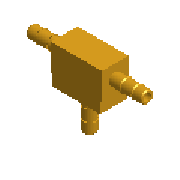
# Autodesk Inventor part: Tubo en T de unión 224 de Parker 224-6
Saved by Autodesk Inventor 2021 (Build 250183000, 183)
## iProperties
NAME: PIPING: Parker Union Tee 224
DATA: <meta><inlinegroups number="1" deflen="2.54"></inlinegroups><connections number="3"></connections><angles><a>3.14159265358979</a><a>1.57079632679489</a></angles></meta>
IsCustomPart: 0
Created: 2020-01-21
Part Number: Tubo en T de unión 224 de Parker 224-6
Material: Latón, amarillo claro
Description: Tubo en T de unión
Document SubType Name: Modeling
Standard: Parker
Designer: Admin
Manufacturer: Parker
Language: es-ES
Size Designation: 224-6
Categories: <MemberInstance><Categories><Category DisplayName="Tubo y tubería" InternalName="4347fa0f-2144-441d-94cd-e3e15c92b736" Mnemonic="TUBEANDPIPE"><CategoryParameter DisplayName="Número de conexiones" InternalName="04e9c83a-9e20-4a98-a7e1-e8abe87a2846" Mnemonic="NUM_CONNECTIONS"/><CategoryParameter DisplayName="Angles" InternalName="0e0e4fa4-3bd3-4656-a22e-4e07c8c476f8" Mnemonic="ANGLES"><CategoryParameter DisplayName="Angle" InternalName="9188ad83-1b16-48b4-8b0a-76ce729dafa7" Mnemonic="ANGLE"/></CategoryParameter><CategoryParameter DisplayName="Angles" InternalName="0e0e4fa4-3bd3-4656-a22e-4e07c8c476f8" Mnemonic="ANGLES"><CategoryParameter DisplayName="Angle" InternalName="9188ad83-1b16-48b4-8b0a-76ce729dafa7" Mnemonic="ANGLE"/></CategoryParameter><CategoryParameter DisplayName="Clave" InternalName="3da84699-049a-4bc2-a65a-6696b77c242f" Mnemonic="SKEY"/><CategoryParameter DisplayName="Descripción ISOGEN" InternalName="7aa3ba45-b821-4467-8584-f9e6f15f2a7d" Mnemonic="ISOGENDESC"/><CategoryParameter DisplayName="CÓDIGO-ARTÍCULO" InternalName="99cc3b15-24d9-4d38-aac7-792cfbc57acf" Mnemonic="ITEMCODE"/><CategoryParameter DisplayName="NombreDeComponente" InternalName="9c74ad13-48a1-45fe-b0f7-5447561f444a" Mnemonic="NAMEOFCOMPONENT"/><CategoryParameter DisplayName="GruposEnLínea" InternalName="d60be647-bc43-4c18-a13f-9fe4115f8e64" Mnemonic="INLINEGROUPS"/><Category DisplayName="Accesorios" InternalName="ed6b26c4-72b8-4f31-9b63-f85ae8f932e4" Mnemonic="FITTINGS"><CategoryParameter DisplayName="Connections" InternalName="dbd721e8-e885-4eea-9011-b5acfd9f61de" Mnemonic="FIT_CONNECTIONS"><CategoryParameter DisplayName="Tamaño de tubería de conicidencia mín." InternalName="11f51b32-3e37-4310-abf7-f1318a1fd129" Mnemonic="MNMPS"/><CategoryParameter DisplayName="EngraneMáx" InternalName="34fdf028-8797-436e-ba07-ca3dee15bd9b" Mnemonic="MAXENGAGEMENT"/><CategoryParameter DisplayName="TamañoNominal" InternalName="3f94edc7-e459-48db-8f02-8eebf8cffccd" Mnemonic="NS"/><CategoryParameter DisplayName="NombreVisualización" InternalName="50f521dd-e050-43f7-9895-6b30ea7ed42e" Mnemonic="DISPLAYNAME"/><CategoryParameter DisplayName="Cortar tubería de coincidencia" InternalName="53a63a6e-53d8-4ca9-8880-037731d1cceb" Mnemonic="CMP"/><CategoryParameter DisplayName="Género neutro" InternalName="628bd5f1-acad-44e2-9d91-af996ab74fc2" Mnemonic="NEUTRAL"/><CategoryParameter DisplayName="EngraneMín [% de EngraneMáx]" InternalName="7ec1bde5-73f0-45b1-98d8-365a6c67f8ad" Mnemonic="MINENGAGEMENT"/><CategoryParameter DisplayName="Fijo" InternalName="9142902a-6a8a-446d-9eb8-4b7ce7d245ef" Mnemonic="FIXED"/><CategoryParameter DisplayName="Hembra" InternalName="b366bcb5-a500-4bad-84bb-22f956216d69" Mnemonic="FEMALE"/><CategoryParameter DisplayName="DirecciónGiro" InternalName="d55dedc0-f14a-4283-86b4-a4eeb253c8aa" Mnemonic="FLIPDIRECTION"/><CategoryParameter DisplayName="NúmeroPlanificación" InternalName="d6161c62-eb59-4495-a086-874847c10866" Mnemonic="SN"/><CategoryParameter DisplayName="TratamientoFinal" InternalName="d7f11516-3374-45ca-b1c7-4b2d63244ae2" Mnemonic="ENDTREATMENT"/><CategoryParameter DisplayName="Tamaño de tubería de conicidencia máx." InternalName="e73ef66b-c04b-45ac-9b32-f712653e25ee" Mnemonic="MXMPS"/></CategoryParameter><CategoryParameter DisplayName="Connections" InternalName="dbd721e8-e885-4eea-9011-b5acfd9f61de" Mnemonic="FIT_CONNECTIONS"><CategoryParameter DisplayName="Tamaño de tubería de conicidencia mín." InternalName="11f51b32-3e37-4310-abf7-f1318a1fd129" Mnemonic="MNMPS"/><CategoryParameter DisplayName="EngraneMáx" InternalName="34fdf028-8797-436e-ba07-ca3dee15bd9b" Mnemonic="MAXENGAGEMENT"/><CategoryParameter DisplayName="TamañoNominal" InternalName="3f94edc7-e459-48db-8f02-8eebf8cffccd" Mnemonic="NS"/><CategoryParameter DisplayName="NombreVisualización" InternalName="50f521dd-e050-43f7-9895-6b30ea7ed42e" Mnemonic="DISPLAYNAME"/><CategoryParameter DisplayName="Cortar tubería de coincidencia" InternalName="53a63a6e-53d8-4ca9-8880-037731d1cceb" Mnemonic="CMP"/><CategoryParameter DisplayName="Género neutro" InternalName="628bd5f1-acad-44e2-9d91-af996ab74fc2" Mnemonic="NEUTRAL"/><CategoryParameter DisplayName="EngraneMín [% de EngraneMáx]" InternalName="7ec1bde5-73f0-45b1-98d8-365a6c67f8ad" Mnemonic="MINENGAGEMENT"/><CategoryParameter DisplayName="Fijo" InternalName="9142902a-6a8a-446d-9eb8-4b7ce7d245ef" Mnemonic="FIXED"/><CategoryParameter DisplayName="Hembra" InternalName="b366bcb5-a500-4bad-84bb-22f956216d69" Mnemonic="FEMALE"/><CategoryParameter DisplayName="DirecciónGiro" InternalName="d55dedc0-f14a-4283-86b4-a4eeb253c8aa" Mnemonic="FLIPDIRECTION"/><CategoryParameter DisplayName="NúmeroPlanificación" InternalName="d6161c62-eb59-4495-a086-874847c10866" Mnemonic="SN"/><CategoryParameter DisplayName="TratamientoFinal" InternalName="d7f11516-3374-45ca-b1c7-4b2d63244ae2" Mnemonic="ENDTREATMENT"/><CategoryParameter DisplayName="Tamaño de tubería de conicidencia máx." InternalName="e73ef66b-c04b-45ac-9b32-f712653e25ee" Mnemonic="MXMPS"/></CategoryParameter><CategoryParameter DisplayName="Connections" InternalName="dbd721e8-e885-4eea-9011-b5acfd9f61de" Mnemonic="FIT_CONNECTIONS"><CategoryParameter DisplayName="Tamaño de tubería de conicidencia mín." InternalName="11f51b32-3e37-4310-abf7-f1318a1fd129" Mnemonic="MNMPS"/><CategoryParameter DisplayName="EngraneMáx" InternalName="34fdf028-8797-436e-ba07-ca3dee15bd9b" Mnemonic="MAXENGAGEMENT"/><CategoryParameter DisplayName="TamañoNominal" InternalName="3f94edc7-e459-48db-8f02-8eebf8cffccd" Mnemonic="NS"/><CategoryParameter DisplayName="NombreVisualización" InternalName="50f521dd-e050-43f7-9895-6b30ea7ed42e" Mnemonic="DISPLAYNAME"/><CategoryParameter DisplayName="Cortar tubería de coincidencia" InternalName="53a63a6e-53d8-4ca9-8880-037731d1cceb" Mnemonic="CMP"/><CategoryParameter DisplayName="Género neutro" InternalName="628bd5f1-acad-44e2-9d91-af996ab74fc2" Mnemonic="NEUTRAL"/><CategoryParameter DisplayName="EngraneMín [% de EngraneMáx]" InternalName="7ec1bde5-73f0-45b1-98d8-365a6c67f8ad" Mnemonic="MINENGAGEMENT"/><CategoryParameter DisplayName="Fijo" InternalName="9142902a-6a8a-446d-9eb8-4b7ce7d245ef" Mnemonic="FIXED"/><CategoryParameter DisplayName="Hembra" InternalName="b366bcb5-a500-4bad-84bb-22f956216d69" Mnemonic="FEMALE"/><CategoryParameter DisplayName="DirecciónGiro" InternalName="d55dedc0-f14a-4283-86b4-a4eeb253c8aa" Mnemonic="FLIPDIRECTION"/><CategoryParameter DisplayName="NúmeroPlanificación" InternalName="d6161c62-eb59-4495-a086-874847c10866" Mnemonic="SN"/><CategoryParameter DisplayName="TratamientoFinal" InternalName="d7f11516-3374-45ca-b1c7-4b2d63244ae2" Mnemonic="ENDTREATMENT"/><CategoryParameter DisplayName="Tamaño de tubería de conicidencia máx." InternalName="e73ef66b-c04b-45ac-9b32-f712653e25ee" Mnemonic="MXMPS"/></CategoryParameter><Category DisplayName="Tubos en T" InternalName="63457372-9f68-4568-9fa2-68fa0de1b1dd" Mnemonic="Tee"/></Category></Category><Category DisplayName="TipoDatos" InternalName="23b78d0f-2648-40c6-8793-ca6db495c9e8" Mnemonic="DATATYPE"><CategoryParameter DisplayName="NombreVisualización" InternalName="05415f3d-3907-474b-a020-eb9d644f4cf3" Mnemonic="DISPLAYNAME"/><CategoryParameter DisplayName="Estándar" InternalName="0c0a119c-1e12-4c84-803f-101930972f5e" Mnemonic="STANDARD"/><CategoryParameter DisplayName="Descripción" InternalName="13903e3d-64b1-4950-80da-f627842ea37f" Mnemonic="DESCRIPTION"/><CategoryParameter DisplayName="Designación" InternalName="2675968c-4ce5-49e0-a4f5-552d29089031" Mnemonic="DESIGNATION"/><CategoryParameter DisplayName="Fila por defecto" InternalName="2af9ec52-faaa-4026-b378-f9fa4afca842" Mnemonic="DEFAULTROW"/><CategoryParameter DisplayName="Nombre de carpeta" InternalName="3f06958e-8713-4116-9be7-ed6184ecc97b" Mnemonic="FOLDERNAME"/><CategoryParameter DisplayName="Guid de revisión" InternalName="45a75005-10b1-4dfc-8d6d-dfe629f0b93c" Mnemonic="REVISIONGUID"/><CategoryParameter DisplayName="NombreArchivo" InternalName="8b46a4cc-9585-4fed-90c3-899f57e09a73" Mnemonic="FILENAME"/><CategoryParameter DisplayName="OrgEstand" InternalName="8f5914e1-4693-403f-8ab5-d37768198c9d" Mnemonic="STDSORG"/><CategoryParameter DisplayName="Versión de familia" InternalName="914462f6-6e19-4b14-ba84-155b9680b1d0" Mnemonic="FAMILYREVISION"/><CategoryParameter DisplayName="Revisión de Norma" InternalName="91d5a463-65c2-4fde-b823-3b7fea5e8e17" Mnemonic="STANDARDREVISION"/><CategoryParameter DisplayName="Revisión del miembro" InternalName="a65d44b9-392f-4f4f-857b-e4b3d54996fe" Mnemonic="MEMBERREVISION"/><CategoryParameter DisplayName="FormatoDelimitación" InternalName="bc51e27b-3422-4e78-93ef-cec197ddf230" Mnemonic="CLIPFORMAT"/><CategoryParameter DisplayName="Fabricante" InternalName="cd6c7a72-a28a-4e50-99a9-2c7f4e13e5ad" Mnemonic="MANUFACTURER"/><CategoryParameter DisplayName="NombreInterno" InternalName="cf1d0246-76d9-4b4a-8305-fa0409afb5c1" Mnemonic="INTERNALNAME"/><CategoryParameter DisplayName="EsMétrico" InternalName="e2385c5b-1ea4-4823-96a8-8de651266ec3" Mnemonic="ISMETRIC"/><Category DisplayName="Pieza" InternalName="c0e0b642-3bcb-4cc8-9e80-f96d35c4afa4" Mnemonic="PART"><CategoryParameter DisplayName="Número de pieza" InternalName="016b6077-bfbe-49bd-92c9-d8d59c39c941" Mnemonic="PARTNUMBER"/><CategoryParameter DisplayName="Referencia de almacén" InternalName="4dba7c1c-e26c-444e-836c-b08b433409a8" Mnemonic="STOCKNUMBER"/><CategoryParameter DisplayName="Clave de material" InternalName="5c9a8adb-dd2b-4535-b97f-0a94a95fe41f" Mnemonic="MATERIALKEY"/><CategoryParameter DisplayName="Material" InternalName="818a152a-d3c3-49ca-80ee-df7d91421b8e" Mnemonic="MATERIAL"/></Category></Category><Category DisplayName="AsignaciónHeredada" InternalName="dfeab48a-acc2-4514-a11c-1b8dc28c3d5f" Mnemonic="LEGACYMAP"><CategoryParameter DisplayName="IDCatálogo" InternalName="0da51c36-8fd3-4028-86cc-0c9c9e96136a" Mnemonic="CATALOGID"/><CategoryParameter DisplayName="IDFamilia" InternalName="1c0b589c-8bbe-4e1e-80cf-07c0de42ac2a" Mnemonic="FAMILYID"/><CategoryParameter DisplayName="IDMiembro" InternalName="a368ea03-db8a-4d6e-962b-2aa46306b8f5" Mnemonic="MEMBERID"/></Category></Categories><FamilyTemplate Id="Parker Union Tee 224"><FamilyTemplateParameters><FamilyTemplateParameter ObjectType="kUserParameterObject" ValueType="xs:double" Id="1" ObjectReferenceKey="L"/><FamilyTemplateParameter ObjectType="kUserParameterObject" ValueType="xs:double" Id="2" ObjectReferenceKey="M"/><FamilyTemplateParameter ObjectType="kUserParameterObject" ValueType="xs:double" Id="3" ObjectReferenceKey="D"/><FamilyTemplateParameter ObjectType="kUserParameterObject" ValueType="xs:double" Id="4" ObjectReferenceKey="D1"/><FamilyTemplateParameter ObjectType="kUserParameterObject" ValueType="xs:double" Id="5" ObjectReferenceKey="D2"/><FamilyTemplateParameter ObjectType="kUserParameterObject" ValueType="xs:double" Id="6" ObjectReferenceKey="L1"/><FamilyTemplateParameter ObjectType="kUserParameterObject" ValueType="xs:double" Id="7" ObjectReferenceKey="L2"/><FamilyTemplateParameter ObjectType="kUserParameterObject" ValueType="xs:double" Id="8" ObjectReferenceKey="L3"/><FamilyTemplateParameter ObjectType="kUserParameterObject" ValueType="xs:double" Id="9" ObjectReferenceKey="W1"/><FamilyTemplateParameter ObjectType="kUserParameterObject" ValueType="xs:string" Id="120" ObjectReferenceKey="Parker_No"/><FamilyTemplateParameter ObjectType="kPropertyObject" ValueType="xs:string" Id="100" ObjectReferenceKey="{32853F0F-3444-11d1-9E93-0060B03C1CA6}" SubObjectId="52"/><FamilyTemplateParameter ObjectType="kPropertyObject" ValueType="xs:string" Id="105" ObjectReferenceKey="{32853F0F-3444-11d1-9E93-0060B03C1CA6}" SubObjectId="5"/><FamilyTemplateParameter ObjectType="kPartComponentDefinitionObject" ValueType="xs:string" Id="110" SubObjectId="Material"/></FamilyTemplateParameters></FamilyTemplate><CategoryParameterMap><ParamToTemplateMap><ParamToTemplate CategoryParameter="//CategoryParameter[@InternalName='d60be647-bc43-4c18-a13f-9fe4115f8e64']" ConstantValue="1"/><ParamToTemplate CategoryParameter="//CategoryParameter[@InternalName='04e9c83a-9e20-4a98-a7e1-e8abe87a2846']" ConstantValue="3"/><ParamToTemplate CategoryParameter="//CategoryParameter[@InternalName='0e0e4fa4-3bd3-4656-a22e-4e07c8c476f8']" ConstantValue=""/><ParamToTemplate CategoryParameter="//CategoryParameter[@InternalName='0e0e4fa4-3bd3-4656-a22e-4e07c8c476f8'][1]/CategoryParameter[@InternalName='9188ad83-1b16-48b4-8b0a-76ce729dafa7']" ConstantValue="3.14159265358979"/><ParamToTemplate CategoryParameter="//CategoryParameter[@InternalName='0e0e4fa4-3bd3-4656-a22e-4e07c8c476f8'][2]/CategoryParameter[@InternalName='9188ad83-1b16-48b4-8b0a-76ce729dafa7']" ConstantValue="1.57079632679489"/><ParamToTemplate CategoryParameter="//CategoryParameter[@InternalName='9c74ad13-48a1-45fe-b0f7-5447561f444a']" ConstantValue="TEE"/><ParamToTemplate CategoryParameter="//CategoryParameter[@InternalName='3da84699-049a-4bc2-a65a-6696b77c242f']" ConstantValue="TECP"/><ParamToTemplate CategoryParameter="//CategoryParameter[@InternalName='dbd721e8-e885-4eea-9011-b5acfd9f61de'][1]/CategoryParameter[@InternalName='d55dedc0-f14a-4283-86b4-a4eeb253c8aa']" ConstantValue="true"/><ParamToTemplate CategoryParameter="//CategoryParameter[@InternalName='dbd721e8-e885-4eea-9011-b5acfd9f61de'][1]/CategoryParameter[@InternalName='50f521dd-e050-43f7-9895-6b30ea7ed42e']" ConstantValue="Connection1"/><ParamToTemplate CategoryParameter="//CategoryParameter[@InternalName='dbd721e8-e885-4eea-9011-b5acfd9f61de'][1]/CategoryParameter[@InternalName='b366bcb5-a500-4bad-84bb-22f956216d69']" ConstantValue="false"/><ParamToTemplate CategoryParameter="//CategoryParameter[@InternalName='dbd721e8-e885-4eea-9011-b5acfd9f61de'][1]/CategoryParameter[@InternalName='d7f11516-3374-45ca-b1c7-4b2d63244ae2']" ConstantValue="Quick Connection"/><ParamToTemplate CategoryParameter="//CategoryParameter[@InternalName='dbd721e8-e885-4eea-9011-b5acfd9f61de'][1]/CategoryParameter[@InternalName='9142902a-6a8a-446d-9eb8-4b7ce7d245ef']" ConstantValue="false"/><ParamToTemplate CategoryParameter="//CategoryParameter[@InternalName='dbd721e8-e885-4eea-9011-b5acfd9f61de'][1]/CategoryParameter[@InternalName='34fdf028-8797-436e-ba07-ca3dee15bd9b']" ConstantValue="0"/><ParamToTemplate CategoryParameter="//CategoryParameter[@InternalName='dbd721e8-e885-4eea-9011-b5acfd9f61de'][1]/CategoryParameter[@InternalName='7ec1bde5-73f0-45b1-98d8-365a6c67f8ad']" ConstantValue="50"/><ParamToTemplate CategoryParameter="//CategoryParameter[@InternalName='dbd721e8-e885-4eea-9011-b5acfd9f61de'][2]/CategoryParameter[@InternalName='d55dedc0-f14a-4283-86b4-a4eeb253c8aa']" ConstantValue="false"/><ParamToTemplate CategoryParameter="//CategoryParameter[@InternalName='dbd721e8-e885-4eea-9011-b5acfd9f61de'][2]/CategoryParameter[@InternalName='50f521dd-e050-43f7-9895-6b30ea7ed42e']" ConstantValue="Connection2"/><ParamToTemplate CategoryParameter="//CategoryParameter[@InternalName='dbd721e8-e885-4eea-9011-b5acfd9f61de'][2]/CategoryParameter[@InternalName='b366bcb5-a500-4bad-84bb-22f956216d69']" ConstantValue="false"/><ParamToTemplate CategoryParameter="//CategoryParameter[@InternalName='dbd721e8-e885-4eea-9011-b5acfd9f61de'][2]/CategoryParameter[@InternalName='d7f11516-3374-45ca-b1c7-4b2d63244ae2']" ConstantValue="Quick Connection"/><ParamToTemplate CategoryParameter="//CategoryParameter[@InternalName='dbd721e8-e885-4eea-9011-b5acfd9f61de'][2]/CategoryParameter[@InternalName='9142902a-6a8a-446d-9eb8-4b7ce7d245ef']" ConstantValue="false"/><ParamToTemplate CategoryParameter="//CategoryParameter[@InternalName='dbd721e8-e885-4eea-9011-b5acfd9f61de'][2]/CategoryParameter[@InternalName='34fdf028-8797-436e-ba07-ca3dee15bd9b']" ConstantValue="0"/><ParamToTemplate CategoryParameter="//CategoryParameter[@InternalName='dbd721e8-e885-4eea-9011-b5acfd9f61de'][2]/CategoryParameter[@InternalName='7ec1bde5-73f0-45b1-98d8-365a6c67f8ad']" ConstantValue="50"/><ParamToTemplate CategoryParameter="//CategoryParameter[@InternalName='dbd721e8-e885-4eea-9011-b5acfd9f61de'][3]/CategoryParameter[@InternalName='d55dedc0-f14a-4283-86b4-a4eeb253c8aa']" ConstantValue="false"/><ParamToTemplate CategoryParameter="//CategoryParameter[@InternalName='dbd721e8-e885-4eea-9011-b5acfd9f61de'][3]/CategoryParameter[@InternalName='50f521dd-e050-43f7-9895-6b30ea7ed42e']" ConstantValue="Connection3"/><ParamToTemplate CategoryParameter="//CategoryParameter[@InternalName='dbd721e8-e885-4eea-9011-b5acfd9f61de'][3]/CategoryParameter[@InternalName='b366bcb5-a500-4bad-84bb-22f956216d69']" ConstantValue="false"/><ParamToTemplate CategoryParameter="//CategoryParameter[@InternalName='dbd721e8-e885-4eea-9011-b5acfd9f61de'][3]/CategoryParameter[@InternalName='d7f11516-3374-45ca-b1c7-4b2d63244ae2']" ConstantValue="Quick Connection"/><ParamToTemplate CategoryParameter="//CategoryParameter[@InternalName='dbd721e8-e885-4eea-9011-b5acfd9f61de'][3]/CategoryParameter[@InternalName='9142902a-6a8a-446d-9eb8-4b7ce7d245ef']" ConstantValue="false"/><ParamToTemplate CategoryParameter="//CategoryParameter[@InternalName='dbd721e8-e885-4eea-9011-b5acfd9f61de'][3]/CategoryParameter[@InternalName='34fdf028-8797-436e-ba07-ca3dee15bd9b']" ConstantValue="0"/><ParamToTemplate CategoryParameter="//CategoryParameter[@InternalName='dbd721e8-e885-4eea-9011-b5acfd9f61de'][3]/CategoryParameter[@InternalName='7ec1bde5-73f0-45b1-98d8-365a6c67f8ad']" ConstantValue="50"/><ParamToTemplate CategoryParameter="//CategoryParameter[@InternalName='05415f3d-3907-474b-a020-eb9d644f4cf3']" ConstantValue="Parker Union Tee 224"/><ParamToTemplate CategoryParameter="//CategoryParameter[@InternalName='cf1d0246-76d9-4b4a-8305-fa0409afb5c1']" ConstantValue="2270a981-9f5a-4234-b233-e648020e18ae"/><ParamToTemplate CategoryParameter="//CategoryParameter[@InternalName='3f06958e-8713-4116-9be7-ed6184ecc97b']" ConstantValue="Parker U T 224"/><ParamToTemplate CategoryParameter="//CategoryParameter[@InternalName='914462f6-6e19-4b14-ba84-155b9680b1d0']" ConstantValue="10"/><ParamToTemplate CategoryParameter="//CategoryParameter[@InternalName='13903e3d-64b1-4950-80da-f627842ea37f']" ConstantValue="Union Tee"/><ParamToTemplate CategoryParameter="//CategoryParameter[@InternalName='8f5914e1-4693-403f-8ab5-d37768198c9d']" TemplateParameter="101"/><ParamToTemplate CategoryParameter="//CategoryParameter[@InternalName='0c0a119c-1e12-4c84-803f-101930972f5e']" ConstantValue="Parker"/><ParamToTemplate CategoryParameter="//CategoryParameter[@InternalName='cd6c7a72-a28a-4e50-99a9-2c7f4e13e5ad']" ConstantValue="Parker"/><ParamToTemplate CategoryParameter="//CategoryParameter[@InternalName='91d5a463-65c2-4fde-b823-3b7fea5e8e17']" TemplateParameter="103"/><ParamToTemplate CategoryParameter="//CategoryParameter[@InternalName='bc51e27b-3422-4e78-93ef-cec197ddf230']" ConstantValue="CF_INVENTOR.STDPARTS"/><ParamToTemplate CategoryParameter="//CategoryParameter[@InternalName='e2385c5b-1ea4-4823-96a8-8de651266ec3']" ConstantValue="false"/><ParamToTemplate CategoryParameter="//CategoryParameter[@InternalName='45a75005-10b1-4dfc-8d6d-dfe629f0b93c']" ConstantValue="cb4cb7d0-872c-47ab-814c-3fec262e9b10"/><ParamToTemplate CategoryParameter="//CategoryParameter[@InternalName='2af9ec52-faaa-4026-b378-f9fa4afca842']" ConstantValue="1"/><ParamToTemplate CategoryParameter="//CategoryParameter[@InternalName='0da51c36-8fd3-4028-86cc-0c9c9e96136a']" ConstantValue="FD8AAA93-B897-476C-BD5D-67C712EC5ABF"/><ParamToTemplate CategoryParameter="//CategoryParameter[@InternalName='1c0b589c-8bbe-4e1e-80cf-07c0de42ac2a']" ConstantValue="2270a981-9f5a-4234-b233-e648020e18ae"/><ParamToTemplate CategoryParameter="//CategoryParameter[@InternalName='99cc3b15-24d9-4d38-aac7-792cfbc57acf']" ConstantValue=""/><ParamToTemplate CategoryParameter="//CategoryParameter[@InternalName='7aa3ba45-b821-4467-8584-f9e6f15f2a7d']" ConstantValue=""/><ParamToTemplate CategoryParameter="//CategoryParameter[@InternalName='dbd721e8-e885-4eea-9011-b5acfd9f61de'][1]/CategoryParameter[@InternalName='3f94edc7-e459-48db-8f02-8eebf8cffccd']" ConstantValue="3/8"/><ParamToTemplate CategoryParameter="//CategoryParameter[@InternalName='dbd721e8-e885-4eea-9011-b5acfd9f61de'][2]/CategoryParameter[@InternalName='3f94edc7-e459-48db-8f02-8eebf8cffccd']" ConstantValue="3/8"/><ParamToTemplate CategoryParameter="//CategoryParameter[@InternalName='dbd721e8-e885-4eea-9011-b5acfd9f61de'][3]/CategoryParameter[@InternalName='3f94edc7-e459-48db-8f02-8eebf8cffccd']" ConstantValue="3/8"/><ParamToTemplate CategoryParameter="//CategoryParameter[@InternalName='8b46a4cc-9585-4fed-90c3-899f57e09a73']" ConstantValue="Tubo en T de unión 224 de Parker 224-6"/><ParamToTemplate CategoryParameter="//CategoryParameter[@InternalName='a65d44b9-392f-4f4f-857b-e4b3d54996fe']" ConstantValue="c2a0cd4d-b98e-4638-9045-95679a552341"/><ParamToTemplate CategoryParameter="//CategoryParameter[@InternalName='a368ea03-db8a-4d6e-962b-2aa46306b8f5']" ConstantValue="688134EB-B09A-4096-A06D-D18F24FBDE48"/><ParamToTemplate CategoryParameter="//CategoryParameter[@InternalName='2675968c-4ce5-49e0-a4f5-552d29089031']" TemplateParameter="100"/><ParamToTemplate CategoryParameter="//CategoryParameter[@InternalName='818a152a-d3c3-49ca-80ee-df7d91421b8e']" TemplateParameter="110"/><ParamToTemplate CategoryParameter="//CategoryParameter[@InternalName='016b6077-bfbe-49bd-92c9-d8d59c39c941']" TemplateParameter="105"/></ParamToTemplateMap></CategoryParameterMap></MemberInstance>
Density: 8.47 g/cm^3
Appearance: Latón - Satinado
Author: Admin
Autodesk Inventor part; units mm, degrees
ref_plane "YZ Plane" through (0, 0, 0) normal (1, 0, 0) x (0, 1, 0)
ref_plane "XZ Plane" through (0, 0, 0) normal (0, 1, 0) x (-1, 0, 0)
ref_plane "XY Plane" through (0, 0, 0) normal (0, 0, 1) x (1, 0, 0)
sketch "Sketch7" plane through (0, 0, 0) normal (0, 0, 1) x (1, 0, 0)
  line L0 (0, 21.209) -> (11.3919, 21.209)
  line L1 (11.3919, 21.209) -> (11.3919, 21.209)
  line L2 (11.3919, 21.209) -> (23.6601, 21.209)
  line L3 (23.6601, 21.209) -> (23.6601, 21.209)
  line L4 (23.6601, 21.209) -> (35.052, 21.209)
  line L5 (35.052, 21.209) -> (35.052, 17.526)
  line L6 (0, 17.526) -> (0, 21.209)
  line L7 (0, 17.526) -> (35.052, 17.526)
  line L8 (-6.2642, 17.526) -> (48.9647, 17.526)
  point P0 (0, 0)
  dimension "d57" = 17.526
  dimension "d58" = 7.366
  dimension "d59" = 35.052
  dimension "d60" = 12.2682
  dimension "d128" = 3.683
  constraints: 18 end point, 5 collinear, 3 parallel, 2 perpendicular, 2 point on line, 1 horizontal
  measures "d57" distance from line of point (0, 0) L7
  measures "d58" diameter of L0 L8
  measures "d59" distance between parallel lines of L5 L6
  measures "d60" distance of L1.end L2.end
  measures "d128" distance between parallel lines of L7 L2
revolve "Revolution3" add sketch "Sketch7" angle 360 about axis through (-6.2642, 17.526, 0) along (1, 0, 0)
ref_plane "Work Plane3" through (17.526, 17.526, 0) normal (-1, 0, 0) x (0, 0, 1)
sketch "Sketch8" plane through (17.526, 17.526, 0) normal (-1, 0, 0) x (0, 0, 1)
  line L0 (-4.064, 4.064) -> (4.064, 4.064)
  line L1 (4.064, 4.064) -> (4.064, -4.064)
  line L2 (4.064, -4.064) -> (-4.064, -4.064)
  line L3 (-4.064, -4.064) -> (-4.064, 4.064)
  circle A0 centre (0, 0) radius 1.3335
  circle A1 centre (0, 0) radius 3.683 projected
  dimension "d119" = 8.128
  dimension "d121" = 8.128
  dimension "d129" = 4.064
  dimension "d130" = 4.064
  constraints: 8 end point, 2 parallel, 1 centre point, 1 concentric, 1 horizontal, 1 perpendicular
  measures "d119" distance between parallel lines of L1 L3
  measures "d121" distance between parallel lines of L0 L2
  measures "d129" distance from line of L2 A0.centre
  measures "d130" distance from line of A0.centre L3
extrude "Extrusion5" add sketch "Sketch8" against normal mid plane 12.2936 contours L0 L1 L2 L3 | A1
sketch "Sketch9" plane through (0, 0, 0) normal (0, 0, 1) x (1, 0, 0)
  line L0 (17.526, 15.4328) -> (17.526, -3.476)
  line L1 (11.3792, 13.462) -> (23.6728, 13.462) projected
  line L2 (17.526, 13.462) -> (21.2458, 13.462)
  line L3 (21.2458, 13.462) -> (21.2458, 9.9568)
  line L4 (21.2458, 9.9568) -> (21.209, 9.9568)
  line L5 (21.209, 9.9568) -> (21.209, 0)
  line L6 (21.209, 0) -> (17.526, 0)
  line L7 (17.526, 0) -> (17.526, 13.462)
  point P0 (0, 0)
  dimension "d65" = 17.526
  dimension "d66" = 7.366
  dimension "d67" = 7.4397
  dimension "d68" = 3.5052
  constraints: 14 end point, 4 point on line, 3 perpendicular, 1 parallel, 1 vertical
  measures "d65" distance from line of point (0, 0) L0
  measures "d66" diameter of L5 L0
  measures "d67" diameter of L3 L0
  measures "d68" distance of L2.end L3.end
revolve "Revolution4" add sketch "Sketch9" angle 360 about axis through (17.526, 15.4328, 0) along (0, -1, 0)
sketch "Sketch10" plane through (17.526, 9.9568, 0) normal (0, -1, 0) x (1, 0, 0)
  circle A0 centre (0, 0) radius 3.7198 projected
  line L0 (-5.5778, 4.064) -> (5.5778, 4.064)
  line L1 (5.5778, 4.064) -> (5.5778, -4.064)
  line L2 (5.5778, -4.064) -> (-5.5778, -4.064)
  line L3 (-5.5778, -4.064) -> (-5.5778, 4.064)
  line L4 (-6.1468, 4.064) -> (6.1468, 4.064) projected
  line L5 (-6.1468, -4.064) -> (6.1468, -4.064) projected
  line L6 (-17.526, -3.683) -> (-17.526, 3.683) projected
  line L7 (17.526, -3.683) -> (17.526, 3.683) projected
  dimension "d122" = 11.9482
  dimension "d123" = 11.9482
  constraints: 8 end point, 2 collinear, 2 parallel, 1 horizontal, 1 perpendicular
  measures "d122" distance between parallel lines of L6 L3
  measures "d123" distance between parallel lines of L7 L1
extrude "Extrusion6" add sketch "Sketch10" against normal up to surface (3.5052 mm away)
sketch "Sketch11" plane through (0, 0, 0) normal (0, 0, 1) x (1, 0, 0)
  line L0 (-6.2642, 17.526) -> (48.9647, 17.526) projected
  line L1 (0, 21.209) -> (11.3792, 21.209) projected
  line L2 (8.128, 21.209) -> (8.128, 21.4122)
  line L3 (8.128, 21.209) -> (7.9248, 21.209)
  line L4 (7.9248, 21.209) -> (8.128, 21.4122)
  line L5 (23.6728, 21.59) -> (23.6728, 13.462) projected
  line L6 (3.81, 21.209) -> (3.81, 21.4122)
  line L7 (3.81, 21.209) -> (3.6068, 21.209)
  line L8 (3.6068, 21.209) -> (3.81, 21.4122)
  line L9 (17.526, 15.4328) -> (17.526, -3.476) projected
  line L10 (26.924, 21.209) -> (26.924, 21.4122)
  line L11 (26.924, 21.209) -> (27.1272, 21.209)
  line L12 (27.1272, 21.209) -> (26.924, 21.4122)
  line L13 (31.242, 21.209) -> (31.242, 21.4122)
  line L14 (31.242, 21.209) -> (31.4452, 21.209)
  line L15 (31.4452, 21.209) -> (31.242, 21.4122)
  line L16 (0, 13.843) -> (0, 21.209) projected
  dimension "d75" = 45
  dimension "d114" = 0.2032
  dimension "d115" = 3.81
  dimension "d116" = 4.318
  constraints: 24 end point, 6 symmetric about line, 2 collinear, 2 parallel, 2 point on line, 2 vertical, 1 other
  measures "d75" angle of L4 L1
  measures "d114" distance from line of L1 L6.end
  measures "d115" distance between parallel lines of L6 L16
  measures "d116" distance between parallel lines of L2 L6
revolve "Revolution5" add sketch "Sketch11" angle 360 about axis through (-6.2642, 17.526, 0) along (1, 0, 0)
sketch "Sketch12" plane through (0, 0, 0) normal (0, 0, 1) x (1, 0, 0)
  line L0 (13.843, 8.4328) -> (13.843, 8.636)
  line L1 (13.843, 8.4328) -> (13.6398, 8.636)
  line L2 (13.6398, 8.636) -> (13.843, 8.636)
  line L3 (17.526, 15.4328) -> (17.526, -3.476) projected
  line L4 (13.843, 9.9568) -> (13.843, 0) projected
  line L5 (11.322, 7.2263) -> (14.078, 7.2263) projected
  line L6 (13.843, 4.1148) -> (13.843, 4.318)
  line L7 (13.843, 4.1148) -> (13.6398, 4.318)
  line L8 (13.6398, 4.318) -> (13.843, 4.318)
  line L9 (13.843, 0) -> (21.209, 0) projected
  dimension "d89" = 45
  dimension "d90" = 45
  dimension "d124" = 0.2032
  dimension "d125" = 4.318
  dimension "d126" = 4.318
  constraints: 12 end point, 2 collinear, 2 perpendicular, 2 vertical, 1 parallel, 1 other
  measures "d89" angle of L1 L0
  measures "d90" angle of L7 L6
  measures "d124" distance from line of L4 L7.end
  measures "d125" distance between parallel lines of L8 L9
  measures "d126" distance between parallel lines of L8 L2
revolve "Revolution6" add sketch "Sketch12" angle 360 about axis through (17.526, 15.4328, 0) along (0, -1, 0)
hole "Hole3" at (35.052, 17.526, 0) direction (-1, 0, 0) diameter 4.7498 end through all
hole "Hole4" at (17.526, 0, 0) direction (0, 1, 0) diameter 4.7498 depth 17.526 tip angle 118
chamfer "Chamfer3" distance 0.3505 angle 30 1 edges at (0, 13.843, 0) measured on face at (1.2023, 21.1613, -0.5908)
chamfer "Chamfer4" distance 0.3505 angle 30 1 edges at (35.052, 13.843, 0) measured on face at (32.6475, 21.1613, -0.5908)
chamfer "Chamfer5" distance 0.3505 angle 30 1 edges at (13.843, 0, 0) measured on face at (21.1971, 2.7432, 0.2964)
fillet "Fillet1" radius 0.5258 2 edges at (11.9482, 13.462, 0) (23.1038, 13.462, 0)
equation "\"d57\" = M"
equation "\"d58\" = D1"
equation "\"d59\" = L"
equation "\"d60\" = 0.35 * L"
equation "\"d128\" = 0.5 * D1"
equation "\"d119\" = W1"
equation "\"d121\" = W1"
equation "\"d129\" = 0.5 * W1"
equation "\"d130\" = 0.5 * W1"
equation "\"d63\" = L - 2 * L3"
equation "\"d65\" = M"
equation "\"d66\" = D1"
equation "\"d67\" = 1.01 * D1"
equation "\"d68\" = 0.285714 * d60"
equation "\"d122\" = 1.05 * L3"
equation "\"d123\" = 1.05 * L3"
equation "\"d70\" = d60"
equation "\"d114\" = D2"
equation "\"d115\" = L1"
equation "\"d116\" = L2"
equation "\"d124\" = D2"
equation "\"d125\" = L2"
equation "\"d126\" = L2"
equation "\"d95\" = D"
equation "\"d104\" = D"
equation "\"d109\" = M"
equation "\"d111\" = 0.01 * L"
equation "\"d112\" = 0.01 * L"
equation "\"d131\" = 0.01 * L"
equation "\"d132\" = 0.01 * L"
equation "\"d134\" = 0.01 * L"
equation "\"d135\" = 0.01 * L"
equation "\"d127\" = 0.015 * L"
equation "\"L\" = 35.052"
equation "\"M\" = 17.526"
equation "\"D\" = 4.7498"
equation "\"d61\" = 1.75 * D"
equation "\"d84\" = 25.4"
equation "\"d85\" = 1.5748"
equation "\"L1\" = 3.81"
equation "\"L2\" = 4.318"
equation "\"L3\" = 11.3792"
equation "\"D1\" = 7.366"
equation "\"D2\" = 0.2032"
equation "\"W1\" = 8.128"
equation "\"d117\" = -0.5 * L"
body "Solid1"
